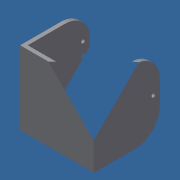
# Autodesk Inventor part: link
Saved by Autodesk Inventor 2014 (Build 180170000, 170)
## iProperties
Created: 2014-04-30
Part Number: link
Material: Generic
Document SubType Name: Modeling
Designer: Lefo
Density: 1 g/cm^3
Appearance: Default
Author: Lefo
Autodesk Inventor part; units mm, degrees
ref_plane "YZ Plane" through (0, 0, 0) normal (1, 0, 0) x (0, 1, 0)
ref_plane "XZ Plane" through (0, 0, 0) normal (0, 1, 0) x (-1, 0, 0)
ref_plane "XY Plane" through (0, 0, 0) normal (0, 0, 1) x (1, 0, 0)
sketch "Sketch1" plane through (0, 0, 0) normal (0, 0, 1) x (1, 0, 0)
  line L0 (-6, 2) -> (-6, 18.7) projected
  line L1 (-29, 18.7) -> (-6, 18.7) projected
  line L2 (-29, 2) -> (-29, 18.7) projected
  line L3 (-6, 2) -> (-29, 2) projected
  line L4 (-47, 5.0995) -> (-47, 15.482) projected
  line L5 (5, 8) -> (5, 13.5) projected
  line L6 (-47, 36.35) -> (5, 36.35)
  line L7 (5, 36.35) -> (5, -15.65)
  line L8 (5, -15.65) -> (-47, -15.65)
  line L9 (-47, -15.65) -> (-47, 36.35)
  line L10 (8, 39.35) -> (-50, 39.35)
  line L11 (-50, 39.35) -> (-50, -18.65)
  line L12 (-50, -18.65) -> (8, -18.65)
  line L13 (8, -18.65) -> (8, 39.35)
  point P0 (0, 0)
  point P1 (-29, 10.35)
  point P2 (-47, 10.35)
  dimension "d0" = 52
  dimension "d1" = 52
  dimension "d2" = 3
  constraints: 16 end point, 4 parallel, 2 collinear, 2 midpoint, 2 perpendicular, 1 horizontal, 1 horizontal alignment, 3 other
  measures "d0" distance of L6.start L6.end
  measures "d1" distance between parallel lines of L8 L6
  measures "d2" distance between parallel lines of L11 L9
extrude "Extrusion1" add sketch "Sketch1" along normal blind 3 contours L3 L2 L1 L0 | L4 L9 L6 L7 L5 L8 | L13 L12 L11 L10
sketch "Sketch2" plane through (0, 0, 0) normal (0, 0, -1) x (-1, 0, 0)
  line L0 (-8, 39.35) -> (50, 39.35) projected
  line L1 (-8, -18.65) -> (-8, 39.35) projected
  line L2 (50, -18.65) -> (-8, -18.65) projected
  line L3 (50, 39.35) -> (50, -18.65) projected
  line L4 (47, 36.35) -> (-5, 36.35)
  line L5 (-5, 36.35) -> (-5, -15.65)
  line L6 (-5, -15.65) -> (47, -15.65)
  line L7 (47, -15.65) -> (47, 36.35)
  line L8 (-5, 36.35) -> (-5, 39.35)
  line L9 (47, 36.35) -> (47, 39.35)
  line L10 (47, -15.65) -> (47, -18.65)
  line L11 (-5, -15.65) -> (-5, -18.65)
  point P0 (0, 0)
  dimension "d5" = 3
  constraints: 16 end point, 4 perpendicular, 4 point on line, 3 other
  measures "d5" distance between parallel lines of L0 L4
extrude "Extrusion2" add sketch "Sketch2" along normal blind 49 contours L0 L8 L5 L11 L2 L1 | L0 L3 L2 L10 L7 L9
sketch "Sketch3" plane through (-50, -18.65, 3) normal (-1, 0, 0) x (0, 0, 1)
  circle A0 centre (-46.753, 29) radius 1.5 projected
  circle A1 centre (-46.6733, 38.9997) radius 1.5 projected
  circle A2 centre (-46.8327, 19.0003) radius 1.5 projected
  point P0 (-3, 18.65)
extrude "Extrusion3" cut sketch "Sketch3" against normal up to next
fillet "Fillet1" radius 20 4 edges at (-48.5, 39.35, -49) (6.5, 39.35, -49) (-48.5, -18.65, -49) (6.5, -18.65, -49)
sketch "Sketch4" plane through (8, -18.65, 3) normal (1, 0, 0) x (0, 0, -1)
  circle A0 centre (46.903, 29.4) radius 2.75 projected
  circle A1 centre (46.903, 29.4) radius 1.5
  point P0 (3, 18.65)
  dimension "d11" = 3
  constraints: 1 centre point, 1 coincident
  measures "d11" diameter of A1
extrude "Extrusion4" cut sketch "Sketch4" against normal up to next contours A1
equation "\"d1\" = d0"
body "Solid1"
